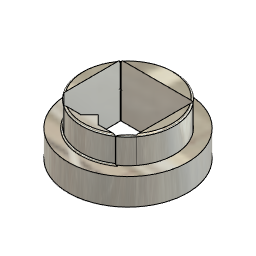
XT30Adaptor (Autodesk Fusion 360 design; units mm, degrees)
Autodesk Fusion 360 part; units mm, degrees
note: some values were not read from the file. Chosen so that the rebuilt part matches the saved one: which bodies a step acts on; which face or edge a step refers to.
sketch "Sketch1" plane through (0, 0, 0) normal (0, 1, 0) x (1, 0, 0)
  circle A0 centre (0, 0) radius 6.5
  line L0 (10.0631, -5.0894) -> (15.2631, -5.0894)
  line L1 (15.2631, -5.0894) -> (15.2631, 5.1106)
  line L2 (15.2631, 5.1106) -> (10.0631, 5.1106)
  line L3 (10.0631, 5.1106) -> (10.0631, -5.0894)
  dimension "d1" = 13
  dimension "d2" = 5.2
  dimension "d3" = 10.2
  constraint coincident A0.centre origin
  constraint horizontal L0
  constraint vertical L1
  constraint horizontal L2
  constraint vertical L3
  measures "d1" diameter of A0
  measures "d2" distance of L0.start L0.end
  measures "d3" distance of L0.start L2.end
sketch "Sketch2" plane through (0, 0, 0) normal (0, 1, 0) x (1, 0, 0)
sketch "Sketch3" plane through (0, 0, 0) normal (0, 1, 0) x (1, 0, 0)
  line L0 (-5.268, 4.2895) -> (-0.068, 4.2895)
  line L1 (-0.068, 4.2895) -> (-0.068, -3.9105)
  line L2 (-0.068, -3.9105) -> (-1.4822, -5.3247)
  line L3 (-0.068, -3.9105) -> (1.932, -3.9105) construction
  line L4 (-1.4822, -5.3247) -> (-3.8322, -5.3247)
  line L5 (-3.8322, -5.3247) -> (-5.2464, -3.9105)
  line L6 (-3.8322, -5.3247) -> (-1.9822, -5.3247) construction
  line L7 (-5.2464, -3.9105) -> (-5.268, 4.2895)
  line L8 (1.3678, -5.3247) -> (-0.0464, -3.9105)
  line L9 (5.132, 4.2895) -> (5.132, -3.9105)
  line L10 (-0.0464, -3.9105) -> (-0.068, 4.2895)
  line L11 (-0.068, 4.2895) -> (5.132, 4.2895)
  line L12 (5.132, -3.9105) -> (3.7178, -5.3247)
  line L13 (3.7178, -5.3247) -> (1.3678, -5.3247)
  line L14 (1.3678, -5.3247) -> (3.2178, -5.3247) construction
  line L15 (-5.2464, -3.9105) -> (5.132, 4.2895)
  line L16 (-5.268, 4.2895) -> (5.132, -3.9105)
  circle A0 centre (-0.068, 0.1895) radius 7
  line L17 (-5.268, 4.2895) -> (5.132, 4.2895)
  line L18 (-0.0464, -3.9105) -> (-0.068, -3.9105)
  circle A1 centre (-0.068, 0.1895) radius 9
  line L19 (-0.0572, -4.324) -> (-1.358, -5.6247)
  line L20 (-1.358, -5.6247) -> (-3.9565, -5.6247)
  line L21 (-3.9565, -5.6247) -> (-5.5461, -4.0351)
  line L22 (-5.5461, -4.0351) -> (-5.5688, 4.5895)
  line L23 (-5.5688, 4.5895) -> (-0.068, 4.5895)
  line L24 (-0.068, 4.5895) -> (5.432, 4.5895)
  line L25 (5.432, 4.5895) -> (5.432, -4.0348)
  line L26 (5.432, -4.0348) -> (3.842, -5.6247)
  line L27 (3.842, -5.6247) -> (1.2435, -5.6247)
  line L28 (1.2435, -5.6247) -> (-0.0572, -4.324)
  dimension "d4" = 5.2
  dimension "d5" = 8.2
  dimension "d6" = 135
  dimension "d7" = 2
  dimension "d8" = 2.35
  dimension "d9" = 135
  dimension "d10" = 2
  dimension "d11" = 5.2
  dimension "d12" = 8.2
  dimension "d13" = 2
  dimension "d14" = 2.35
  dimension "d15" = 135
  dimension "d16" = 2
  dimension "d17" = 14
  dimension "d20" = 18
  dimension "d27" = -0.3
  constraint horizontal L0
  constraint perpendicular L0 L1
  constraint horizontal L3
  constraint perpendicular L1 L4
  constraint horizontal L6
  constraint horizontal L11
  constraint perpendicular L9 L11
  constraint perpendicular L9 L13
  constraint horizontal L14
  constraint midpoint L16 A0.centre
  constraint perpendicular L9 L17
  constraint perpendicular L1 L18
  constraint concentric A0 A1
  measures "d4" distance of L0.start L0.end
  measures "d5" distance of L0.end L1.end
  measures "d6" angle of L2 L3
  measures "d7" distance of L1.end L2.end
  measures "d8" distance of L2.end L4.end
  measures "d9" angle of L5 L6
  measures "d10" distance of L4.end L5.end
  measures "d11" distance of L0.end L9.start
  measures "d12" distance of L9.end L9.start
  measures "d13" distance of L9.end L12.end
  measures "d14" distance of L8.start L12.end
  measures "d15" angle of L8 L14
  measures "d16" distance of L8.start L8.end
  measures "d17" diameter of A0
  measures "d20" diameter of A1
extrude "Extrude1" add sketch "Sketch3" along normal blind 8 contours A0 L25 L26 | A0 L23 L24 | A0 L19 L20 L21 L22 L27 L28 makes body 1 at (-6.295, 5.3333, 3.0082) makes body 2 at (-3.3935, 5.3333, -6.3491) makes body 3 at (5.8347, 2.6667, -3.9522)
extrude "Extrude2" add sketch "Sketch3" along normal blind 4 contours A0 L24 L25 | A0 L26 L27 | A0 L22 L23 | A1 bodies 1
fillet "Fillet1" radius 0.2 1 edges at (-5.2027, 4, 4.5682) on bodies 1
fillet "Fillet2" radius 0.25 3 edges at (-0.068, 8, -7.1895) (-5.2027, 8, 4.5682) (6.8498, 8, 0.8804) on bodies 1 2 3
